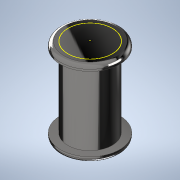
# Autodesk Inventor part: Sketch
Saved by Autodesk Inventor 2020.5 (Build 245400000, 400)
## iProperties
Created: 2020-02-29
Part Number: Sketch
Document SubType Name: Modeling
Designer: Administrator
Density: 7.85 g/cm^3
Material: Acero, alta resistencia, aleación baja
Appearance: Acero - Pulido
Mass: 2.79083 g
Surface Area: 3.59698 cm^2
Volume: 0.35552 cm^3
Author: Administrator
Autodesk Inventor part; units mm, degrees
ref_plane "YZ Plane" through (0, 0, 0) normal (1, 0, 0) x (0, 1, 0)
ref_plane "XZ Plane" through (0, 0, 0) normal (0, 1, 0) x (-1, 0, 0)
ref_plane "XY Plane" through (0, 0, 0) normal (0, 0, 1) x (1, 0, 0)
sketch "Sketch4" plane through (0, 0, 0) normal (1, 0, 0) x (0, 1, 0)
  line L0 (0, 0) -> (3, 0)
  line L1 (3, 0) -> (3, -5)
  line L2 (3, -5) -> (4, -5)
  line L3 (4, -5) -> (4, -5.75)
  line L4 (4, -5.75) -> (0, -5.75)
  line L5 (0, -5.75) -> (0, 0)
  dimension "d32" = 3
  dimension "d33" = 5
  dimension "d35" = 4
  dimension "d36" = 0.75
  constraints: 12 end point, 4 perpendicular, 1 horizontal
  measures "d32" distance between parallel lines of L1 L5
  measures "d33" distance of L0.end L1.end
  measures "d35" distance between parallel lines of L3 L5
  measures "d36" distance of L2.end L3.end
revolve "Revolution2" add sketch "Sketch4" angle 360 about axis through (0, 0, -5.75) along (0, 0, 1)
fillet "Fillet1" radius 0.5 1 edges at (0, -4, -5.75)
mirror "Mirror1" about plane through (0, 3, 0) normal (0, 0, 1) of "Revolution2", "Fillet1"
sketch "Boceto5" plane through (0, 0, 5.75) normal (0, 0, 1) x (1, 0, 0)
  circle A0 centre (0, 0) radius 3 projected
  constraints: 1 coincident
body "Solid4"
